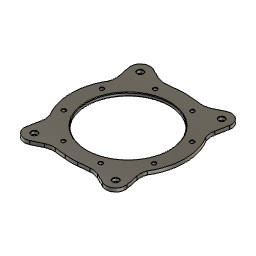
Motor_Base_Plate_Botm v3 (Autodesk Fusion 360 design; units mm, degrees)
Autodesk Fusion 360 part; units mm, degrees
sketch "Sketch1" plane through (0, 0, 0) normal (0, 0, 1) x (1, 0, 0)
  circle A0 centre (0, 0) radius 42.5 construction
  line L0 (0, 0) -> (16.6061, 39.1215) construction
  line L1 (0, 0) -> (42.5, 0) construction
  circle A1 centre (16.6061, 39.1215) radius 1.5
  circle A2 centre (-15.9208, 39.4053) radius 1.5
  circle A3 centre (-39.1215, 16.6061) radius 1.5
  circle A4 centre (-39.4053, -15.9208) radius 1.5
  circle A5 centre (-16.6061, -39.1215) radius 1.5
  circle A6 centre (15.9208, -39.4053) radius 1.5
  circle A7 centre (39.1215, -16.6061) radius 1.5
  circle A8 centre (39.4053, 15.9208) radius 1.5
  circle A9 centre (0, 0) radius 35.5
  line L2 (-49, 64) -> (49, 64) construction
  line L3 (49, 64) -> (49, -64) construction
  line L4 (49, -64) -> (-49, -64) construction
  line L5 (-49, -64) -> (-49, 64) construction
  line L6 (-49, 64) -> (49, -64) construction
  line L7 (49, 64) -> (-49, -64) construction
  line L8 (-41.2883, 33.599) -> (-43.4114, 44.2433)
  arc A10 (-31.5374, 53.3346) -> (-43.4114, 44.2433) centre (-35.1382, 45.7377) ccw
  line L9 (-22.9308, 49.1799) -> (-31.5374, 53.3346)
  arc A11 (-22.9308, 49.1799) -> (-14.9379, 47.7607) centre (-16.4099, 62.6883) ccw
  line L10 (-14.9379, 47.7607) -> (-5.4272, 48.6985)
  arc A12 (-41.9364, 25.3444) -> (-41.2883, 33.599) centre (-55.9855, 30.6002) ccw
  line L11 (0, 2.5) -> (0, 20)
  arc A13 (43.4114, 44.2433) -> (31.5374, 53.3346) centre (35.1382, 45.7377) ccw
  line L12 (22.9308, 49.1799) -> (31.5374, 53.3346)
  arc A14 (14.9379, 47.7607) -> (22.9308, 49.1799) centre (16.4099, 62.6883) ccw
  line L13 (14.9379, 47.7607) -> (5.4272, 48.6985)
  line L14 (41.2883, 33.599) -> (43.4114, 44.2433)
  arc A15 (41.2883, 33.599) -> (41.9364, 25.3444) centre (55.9855, 30.6002) ccw
  line L15 (20, 0) -> (2.5, 0)
  arc A16 (-43.4114, -44.2433) -> (-31.5374, -53.3346) centre (-35.1382, -45.7377) ccw
  line L16 (-22.9308, -49.1799) -> (-31.5374, -53.3346)
  line L17 (-41.2883, -33.599) -> (-43.4114, -44.2433)
  arc A17 (-41.2883, -33.599) -> (-41.9364, -25.3444) centre (-55.9855, -30.6002) ccw
  arc A18 (-14.9379, -47.7607) -> (-22.9308, -49.1799) centre (-16.4099, -62.6883) ccw
  line L18 (-14.9379, -47.7607) -> (-5.4272, -48.6985)
  arc A19 (22.9308, -49.1799) -> (14.9379, -47.7607) centre (16.4099, -62.6883) ccw
  line L19 (14.9379, -47.7607) -> (5.4272, -48.6985)
  line L20 (22.9308, -49.1799) -> (31.5374, -53.3346)
  arc A20 (31.5374, -53.3346) -> (43.4114, -44.2433) centre (35.1382, -45.7377) ccw
  line L21 (41.2883, -33.599) -> (43.4114, -44.2433)
  arc A21 (41.9364, -25.3444) -> (41.2883, -33.599) centre (55.9855, -30.6002) ccw
  circle A22 centre (-35.1382, 45.7377) radius 2.5
  circle A23 centre (35.1382, 45.7377) radius 2.5
  circle A24 centre (-35.1382, -45.7377) radius 2.5
  circle A25 centre (35.1382, -45.7377) radius 2.5
  arc A26 (5.4272, 48.6985) -> (-5.4272, 48.6985) centre (0, 0) ccw
  arc A27 (41.9364, -25.3444) -> (41.9364, 25.3444) centre (0, 0) ccw
  arc A28 (-41.9364, 25.3444) -> (-41.9364, -25.3444) centre (0, 0) ccw
  arc A29 (-5.4272, -48.6985) -> (5.4272, -48.6985) centre (0, 0) ccw
  dimension "d18" = 85
  dimension "d19" = 67
  dimension "d20" = 3
  dimension "d23" = 71
  dimension "d26" = 98
  dimension "d27" = 128
  dimension "d30" = 15
  dimension "d31" = 5
  constraint coincident A0.centre L0.start
  constraint horizontal L1
  constraint coincident A0 L0.end
  constraint coincident L0.end A1.centre
  constraint horizontal L2
  constraint perpendicular L2 L3
  constraint parallel L2 L4
  constraint parallel L3 L5
  constraint coincident L6 A0.centre
  constraint coincident L7 A0.centre
  constraint tangent L5 A28
  constraint tangent L9 A11
  constraint tangent A11 L10
  constraint symmetric A10.start L11 A13.end
  constraint symmetric L9.start L11 L12.start
  constraint symmetric A11.end L11 A14.start
  constraint symmetric L8.end L11 A13.start
  constraint symmetric L8.start L11 L14.start
  constraint symmetric L10.end L11 L13.end
  constraint symmetric A12.start L11 A15.end
  constraint symmetric A10 L11 A13
  constraint symmetric A11 L11 A14
  constraint symmetric A12 L11 A15
  constraint symmetric A10.start L15 A16.end
  constraint symmetric L9.start L15 L16.start
  constraint symmetric A11.end L15 A18.start
  constraint symmetric L8.end L15 A16.start
  constraint symmetric L8.start L15 L17.start
  constraint symmetric L10.end L15 L18.end
  constraint symmetric A12.start L15 A17.end
  constraint symmetric A10 L15 A16
  constraint symmetric A11 L15 A18
  constraint symmetric A12 L15 A17
  constraint symmetric A13.end L15 L20.end
  constraint symmetric A13.start L15 A20.end
  constraint symmetric A13 L15 A20
  constraint symmetric L12.start L15 A19.start
  constraint symmetric A14.start L15 A19.end
  constraint symmetric A14 L15 A19
  constraint symmetric L13.end L15 L19.end
  constraint symmetric L14.start L15 L21.start
  constraint symmetric A15.end L15 A21.start
  constraint symmetric A15 L15 A21
  constraint concentric A10 A22
  constraint symmetric L11 A22 A23
  constraint symmetric L15 A22 A24
  constraint symmetric L15 A23 A25
  constraint concentric A26 A28
  constraint concentric A27 A28
  constraint concentric A28 A29
  measures "d18" diameter of A0
  measures "d19" angle of L0 L1
  measures "d20" diameter of A1
  measures "d23" diameter of A9
  measures "d26" distance of L3.end L4.end
  measures "d27" distance of L2.end L3.end
  measures "d30" radius of A11
  measures "d31" diameter of A22
extrude "Extrude1" add sketch "Sketch1" along normal blind 3
chamfer "Chamfer1" distance 0.5 angle 45 1 faces at (-35.3236, -3.5347, 1)
chamfer "Chamfer1" distance 0.25 angle 45 8 faces at (-38.7152, 15.1621, 1) (-37.9072, -15.9955, 2) (-17.2381, 38.6879, 2) (17.886, 39.9036, 2) (39.8116, 14.4768, 1) (38.4371, -17.9409, 2) (17.2007, -38.6232, 2) (-17.9234, -39.8388, 2)
chamfer "Chamfer1" distance 0.25 angle 45 4 faces at (-36.4946, 43.6376, 2) (-36.4946, -47.8377, 2) (33.7819, -47.8377, 2) (33.7819, 43.6376, 2)
equation "d19 = 90 deg - 23 deg"
